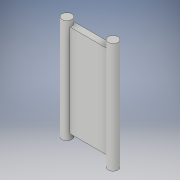
# Autodesk Inventor part: 20_Rect_Aperture_door_slide
Saved by Autodesk Inventor 2019 (Build 230136000, 136)
## iProperties
Created: 2020-03-11
Part Number: 20_Rect_Aperture_door_slide
Material: Generic
Document SubType Name: Modeling
Designer: marsikovabarbora
Density: 1 g/cm^3
Appearance: Default
Author: marsikovabarbora
Autodesk Inventor part; units mm, degrees
ref_plane "YZ Plane" through (0, 0, 0) normal (1, 0, 0) x (0, 1, 0)
sketch "Sketch1" plane through (0, 0, 0) normal (0, 0, 1) x (1, 0, 0)
  line L0 (-9.8, 0) -> (9.8, 0) construction
  line L1 (0, -20.65) -> (0, 20.65) construction
  line L2 (7, -14.75) -> (-7, -14.75)
  line L3 (-7, -14.75) -> (-7, 14.75)
  line L4 (-7, 14.75) -> (7, 14.75)
  line L5 (7, 14.75) -> (7, -14.75)
  line L6 (7, -14.75) -> (-7, 14.75) construction
  line L7 (-7, -14.75) -> (7, 14.75) construction
  point P0 (0, 0)
  dimension "d0" = 14
  dimension "d1" = 29.5
  constraints: 12 end point, 2 midpoint, 2 parallel, 1 horizontal, 1 perpendicular
  measures "d0" distance of L3.end L4.end
  measures "d1" distance of L2.end L3.end
extrude "Extrusion1" add sketch "Sketch1" along normal blind 2
ref_plane "Work Plane1" through (-7, 16.75, 0) normal (0, 1, 0) x (1, 0, 0)
sketch "Sketch2" plane through (-7, 16.75, 0) normal (0, 1, 0) x (1, 0, 0)
  line L0 (0, 0) -> (14, 0) construction
  line L1 (0, 0) -> (0, -2) construction
  line L2 (14, -2) -> (0, -2) construction
  line L3 (14, 0) -> (14, -2) construction
  circle A0 centre (14, -1.5) radius 1.5
  point P0 (7, 0)
  dimension "d5" = 3
  constraints: 1 centre point, 1 point on line, 1 tangent
  measures "d5" diameter of A0
extrude "Extrusion2" add sketch "Sketch2" against normal blind 33.5
ref_plane "Work Plane2" through (-7, 15.75, 2) normal (0, 1, 0) x (1, 0, 0)
sketch "Sketch3" plane through (-7, 15.75, 2) normal (0, 1, 0) x (1, 0, 0)
  arc A0 (14, 2) -> (12.5858, 0) centre (14, 0.5) ccw construction
  line L0 (0, 2) -> (14, 2) construction
  line L1 (0, 2) -> (0, 0) construction
  line L2 (12.5858, 0) -> (0, 0) construction
  line L3 (0, 2) -> (0, 0) projected
  circle A1 centre (0, 0.5) radius 1.5
  point P0 (7, 2)
  dimension "d9" = 3
  constraints: 1 point on line, 1 vertical alignment, 2 other
extrude "Extrusion3" add sketch "Sketch3" against normal blind 31.5
sketch "Skizze5" plane through (-7, 14.75, 0) normal (0, 1, 0) x (1, 0, 0)
  arc A0 (1.4142, -2) -> (0, 0) centre (0, -1.5) ccw projected
  line L0 (12.5858, -2) -> (1.4142, -2) projected
  arc A1 (14, 0) -> (12.5858, -2) centre (14, -1.5) ccw projected
  line L1 (0, 0) -> (14, 0) projected
  point P0 (7, 0)
extrude "Extrusion4" cut sketch "Skizze5" against normal blind 0.75
sketch "Skizze6" plane through (-7, -14.75, 0) normal (0, -1, 0) x (1, 0, 0)
  arc A0 (0, 0) -> (1.4142, 2) centre (0, 1.5) ccw projected
  line L0 (14, 0) -> (0, 0) projected
  arc A1 (12.5858, 2) -> (14, 0) centre (14, 1.5) ccw projected
  line L1 (1.4142, 2) -> (12.5858, 2) projected
  point P0 (7, 0)
extrude "Extrusion5" cut sketch "Skizze6" against normal blind 0.75
equation "\"d6\" = d1 + 2 * d4"
equation "\"d4\" = 2"
body "Solid1"
